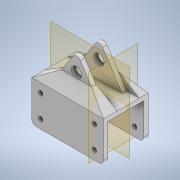
# Autodesk Inventor part: Intake - Piston Mount
Saved by Autodesk Inventor 2020 (Build 240168000, 168)
## iProperties
Created: 2020-02-05
Part Number: Intake - Piston Mount
Material: Generic
Document SubType Name: Modeling
Designer: aidan
Density: 1 g/cm^3
Appearance: Default
Author: aidan
Autodesk Inventor part; units mm, degrees
ref_plane "YZ Plane" through (0, 0, 0) normal (1, 0, 0) x (0, 1, 0)
ref_plane "XZ Plane" through (0, 0, 0) normal (0, 1, 0) x (-1, 0, 0)
ref_plane "XY Plane" through (0, 0, 0) normal (0, 0, 1) x (1, 0, 0)
sketch "Sketch1" plane through (0, 0, 0) normal (0, 1, 0) x (-1, 0, 0)
  line L0 (0, 0) -> (-50.8, 0)
  line L1 (-50.8, 0) -> (-50.8, -25.4)
  line L2 (-50.8, -25.4) -> (0, -25.4)
  line L3 (0, -25.4) -> (0, 0)
  dimension "d0" = 50.8
  dimension "d1" = 25.4
  constraints: 8 end point, 2 parallel, 1 horizontal, 1 perpendicular
  measures "d0" distance of L2.end L1.end
  measures "d1" distance of L1.end L0.end
extrude "Extrusion1" add sketch "Sketch1" along normal blind 3.175
sketch "Sketch2" plane through (0, 3.175, 0) normal (0, 1, 0) x (1, 0, 0)
  line L0 (8.89, 3.175) -> (41.91, 3.175)
  line L1 (41.91, 3.175) -> (41.91, 6.35)
  line L2 (41.91, 6.35) -> (8.89, 6.35)
  line L3 (8.89, 6.35) -> (8.89, 3.175)
  line L4 (8.89, 19.05) -> (41.91, 19.05)
  line L5 (41.91, 19.05) -> (41.91, 22.225)
  line L6 (41.91, 22.225) -> (8.89, 22.225)
  line L7 (8.89, 22.225) -> (8.89, 19.05)
  line L8 (0, 25.4) -> (0, 0) projected
  line L9 (50.8, 0) -> (50.8, 25.4) projected
  line L10 (50.8, 25.4) -> (0, 25.4) projected
  point P0 (41.91, 20.6375)
  point P1 (41.91, 4.7625)
  point P2 (8.89, 20.6375)
  point P3 (8.89, 4.7625)
  dimension "d4" = 8.89
  dimension "d5" = 8.89
  dimension "d6" = 3.175
  dimension "d7" = 12.7
  dimension "d8" = 3.175
  constraints: 16 end point, 4 midpoint, 4 parallel, 2 equal length, 2 horizontal, 2 perpendicular, 2 vertical alignment
  measures "d4" distance between parallel lines of L8 L3
  measures "d5" distance between parallel lines of L9 L1
  measures "d6" distance of L6.end L4.start
  measures "d7" distance between parallel lines of L2 L4
  measures "d8" distance between parallel lines of L10 L6
extrude "Extrusion2" add sketch "Sketch2" along normal blind 38.1
sketch "Sketch3" plane through (8.89, 3.175, -3.175) normal (0, 0, 1) x (1, 0, 0)
  line L0 (0, 0) -> (0, 38.1) projected
  line L1 (0, 0) -> (13.8479, 21.3045)
  line L2 (19.1721, 21.3045) -> (33.02, 0)
  line L3 (33.02, 0) -> (33.02, 38.1) projected
  line L4 (-8.89, 0) -> (41.91, 0) projected
  arc A0 (19.1721, 21.3045) -> (13.8479, 21.3045) centre (16.51, 19.5742) ccw
  line L5 (33.02, 38.1) -> (0, 38.1) projected
  line L6 (0, 38.1) -> (33.02, 38.1)
  point P0 (-8.89, -3.175)
  point P1 (16.51, 25.4)
  dimension "d11" = 25.4
  dimension "d12" = 3.175
  constraints: 6 end point, 4 point on line, 2 point on circle, 2 tangent, 1 centre point, 1 equal length, 1 horizontal
  measures "d11" distance from line of L4 point (16.51, 25.4)
  measures "d12" radius of A0
extrude "Extrusion3" cut sketch "Sketch3" against normal blind 38.1 contours L0 L5 L3 L2 A0 L1
sketch "Sketch4" plane through (8.89, 3.175, -3.175) normal (0, 0, 1) x (1, 0, 0)
  circle A0 centre (16.51, 12.7) radius 3.6539
  line L0 (-8.89, 0) -> (41.91, 0) projected
  point P0 (-8.89, -3.175)
  point P1 (16.51, 0)
  dimension "d15" = 12.7
  constraints: 1 centre point, 1 midpoint, 1 vertical alignment
  measures "d15" distance from line of L0 A0.centre
extrude "Extrusion4" cut sketch "Sketch4" against normal blind 38.1
sketch "Sketch6" plane through (0, 3.175, 0) normal (0, 1, 0) x (1, 0, 0)
  line L0 (50.8, 0) -> (0, 0)
  line L1 (0, 0) -> (0, -3.175)
  line L2 (0, -3.175) -> (50.8, -3.175)
  line L3 (50.8, -3.175) -> (50.8, 0)
  line L4 (50.8, 28.575) -> (0, 28.575)
  line L5 (0, 28.575) -> (0, 25.4)
  line L6 (0, 25.4) -> (50.8, 25.4)
  line L7 (50.8, 25.4) -> (50.8, 28.575)
  line L8 (50.8, 0) -> (50.8, 25.4) projected
  line L9 (0, 25.4) -> (0, 0) projected
  point P0 (50.8, -1.5875)
  point P1 (50.8, 26.9875)
  point P2 (0, -1.5875)
  point P3 (0, 26.9875)
  point P4 (25.4, 0)
  point P5 (0, 12.7)
  dimension "d26" = 0
  dimension "d27" = 3.175
  constraints: 16 end point, 6 midpoint, 4 parallel, 3 vertical alignment, 2 horizontal, 2 perpendicular, 1 coincident, 1 collinear, 1 horizontal alignment
  measures "d26" distance between parallel lines of L8 L3
  measures "d27" distance of L6.end L4.start
extrude "Extrusion5" add sketch "Sketch6" against normal blind 28.575 contours L3 L2 L1 L0 | L6 L5 L4 L7
sketch "Sketch7" plane through (0, 3.175, 3.175) normal (0, 0, 1) x (1, 0, 0)
  line L0 (0, 0) -> (50.8, 0) construction
  line L1 (0, 0) -> (0, -28.575) construction
  line L2 (50.8, -28.575) -> (0, -28.575) construction
  line L3 (50.8, 0) -> (50.8, -28.575) construction
  line L4 (44.45, -22.225) -> (6.35, -22.225) construction
  line L5 (6.35, -22.225) -> (6.35, -6.35) construction
  line L6 (6.35, -6.35) -> (44.45, -6.35) construction
  line L7 (44.45, -6.35) -> (44.45, -22.225) construction
  point P0 (0, -3.175)
  dimension "d30" = 6.35
  constraints: 8 end point, 3 other
  measures "d30" distance between parallel lines of L3 L7
hole "Hole2" at (6.35, -3.175, 3.175) at (44.45, -3.175, 3.175) at (44.45, -19.05, 3.175) at (6.35, -19.05, 3.175) direction (0, 0, -1) diameter 3.175 end through all
fillet "Fillet1" radius 3.175 4 edges at (0, -25.4, 1.5875) (0, -25.4, -26.9875) (50.8, -25.4, 1.5875) (50.8, -25.4, -26.9875)
ref_plane "Work Plane1" through (8.89, 3.175, -12.7) normal (0, 0, 1) x (1, 0, 0)
ref_plane "Work Plane2" through (41.91, 3.175, -3.175) normal (1, 0, 0) x (0, 0, -1)
sketch "Sketch8" plane through (41.91, 3.175, -3.175) normal (1, 0, 0) x (0, 0, -1)
  line L0 (0, 0) -> (0, 9.0461)
  line L1 (-6.35, 0) -> (-6.35, -25.4) projected
  line L2 (0, 9.0461) -> (-6.35, 0)
  line L3 (-6.35, 0) -> (0, 0)
  line L4 (0, 9.0461) -> (0, 16.3539) projected
  point P0 (-3.175, -3.175)
  constraints: 6 end point, 1 perpendicular, 1 vertical
extrude "Extrusion6" add sketch "Sketch8" along normal blind 8.89 and the other way blind 41.91
sketch "Sketch10" plane through (14.7699, 12.2211, -3.175) normal (0, 0, -1) x (-1, 0, 0)
  line L0 (-27.1401, -9.0461) -> (-21.2601, 0) projected
  line L1 (-21.2601, 0) -> (-36.0301, -9.0461)
  line L2 (-36.0301, 0) -> (-36.0301, -9.0461) projected
  line L3 (-21.2601, 0) -> (-36.0301, 0)
  line L4 (-36.0301, -9.0461) -> (-36.0301, 0) projected
  line L5 (-36.0301, 0) -> (-36.0301, -9.0461)
  line L6 (0, 0) -> (5.8799, -9.0461) projected
  line L7 (0, 0) -> (14.7699, -9.0461)
  line L8 (14.7699, -9.0461) -> (14.7699, 0) projected
  line L9 (14.7699, -9.0461) -> (14.7699, 0)
  line L10 (14.7699, 0) -> (0, 0)
  point P0 (14.7699, -12.2211)
  constraints: 12 end point, 2 collinear, 1 horizontal, 1 perpendicular, 1 point on line
extrude "Extrusion8" cut sketch "Sketch10" against normal blind 8.89
mirror "Mirror2" about plane through (8.89, 3.175, -12.7) normal (0, 0, 1) of "Extrusion6", "Extrusion8"
sketch "Sketch11" plane through (8.89, 3.175, -3.175) normal (0, 0, -1) x (-1, 0, 0)
  line L0 (8.89, 0) -> (-5.8799, 9.0461) projected
  line L1 (-5.8799, 9.0461) -> (0, 0) projected
  line L2 (8.89, 0) -> (0, 0) projected
  line L3 (-27.1401, 9.0461) -> (-41.91, 0) projected
  line L4 (-33.02, 0) -> (-41.91, 0) projected
  line L5 (-33.02, 0) -> (-27.1401, 9.0461) projected
  point P0 (8.89, -3.175)
extrude "Extrusion9" add sketch "Sketch11" along normal blind 3.175
body "Solid1"
